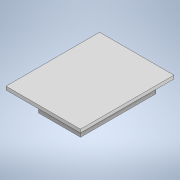
# Autodesk Inventor part: LCDScreen
Saved by Autodesk Inventor 2020 (Build 240168000, 168)
## iProperties
Created: 2019-07-11
Part Number: LCDScreen
Material: Generic
Document SubType Name: Modeling
Designer: El-KhouryJonathan
Density: 1 g/cm^3
Appearance: Default
Author: El-KhouryJonathan
Autodesk Inventor part; units mm, degrees
ref_plane "YZ Plane" through (0, 0, 0) normal (1, 0, 0) x (0, 1, 0)
ref_plane "XZ Plane" through (0, 0, 0) normal (0, 1, 0) x (-1, 0, 0)
ref_plane "XY Plane" through (0, 0, 0) normal (0, 0, 1) x (1, 0, 0)
sketch "Sketch1" plane through (0, 0, 0) normal (0, 1, 0) x (-1, 0, 0)
  point P0 (0, 0)
sketch "Sketch2" plane through (0, 0, 0) normal (0, 1, 0) x (-1, 0, 0)
  line L0 (-139.5, 175.3) -> (139.5, 175.3)
  line L1 (139.5, 175.3) -> (139.5, -175.3)
  line L2 (139.5, -175.3) -> (-139.5, -175.3)
  line L3 (-139.5, -175.3) -> (-139.5, 175.3)
  line L4 (-139.5, 175.3) -> (139.5, -175.3) construction
  line L5 (139.5, 175.3) -> (-139.5, -175.3) construction
  point P0 (0, 0)
  dimension "d0" = 350.6
  dimension "d1" = 279
  constraints: 12 end point, 2 midpoint, 2 parallel, 1 horizontal, 1 perpendicular
  measures "d0" distance of L0.end L1.end
  measures "d1" distance of L0.start L0.end
extrude "Extrusion1" add sketch "Sketch2" along normal blind 12.4
sketch "Sketch3" plane through (0, 0, 0) normal (0, -1, 0) x (1, 0, 0)
  line L0 (-125.5, -159.875) -> (125.5, -159.875)
  line L1 (125.5, -159.875) -> (125.5, 159.875)
  line L2 (125.5, 159.875) -> (-125.5, 159.875)
  line L3 (-125.5, 159.875) -> (-125.5, -159.875)
  line L4 (-125.5, -159.875) -> (125.5, 159.875) construction
  line L5 (125.5, -159.875) -> (-125.5, 159.875) construction
  point P0 (0, 0)
  dimension "d4" = 319.75
  dimension "d5" = 251
  constraints: 12 end point, 2 midpoint, 2 parallel, 1 horizontal, 1 perpendicular
  measures "d4" distance of L2.end L0.start
  measures "d5" distance of L1.end L2.end
extrude "Extrusion2" add sketch "Sketch3" along normal blind 13.5
sketch "Sketch4" plane through (0, -13.5, 0) normal (0, -1, 0) x (1, 0, 0)
  line L0 (125.5, 159.875) -> (-125.5, 159.875) projected
  line L1 (-125.5, 159.875) -> (-125.5, -159.875) projected
  line L2 (125.5, -159.875) -> (125.5, 159.875) projected
  line L3 (-125.5, -159.875) -> (125.5, -159.875) projected
  point P0 (0, 0)
  point P1 (-115.5, 149.875)
  point P2 (-115.5, -149.875)
  point P3 (115.5, 149.875)
  point P4 (115.5, -149.875)
  dimension "d15" = 10
  dimension "d16" = 10
  dimension "d19" = 299.75
  dimension "d22" = 231
  dimension "d25" = 10
  dimension "d26" = 10
  constraints: 1 horizontal, 1 vertical, 3 other
  measures "d15" distance from line of L0 point (-115.5, 149.875)
  measures "d16" distance from line of L1 point (-115.5, 149.875)
  measures "d19" distance of point (-115.5, 149.875) point (-115.5, -149.875)
  measures "d22" distance of point (-115.5, 149.875) point (115.5, 149.875)
  measures "d25" distance from line of L2 point (115.5, 149.875)
  measures "d26" distance from line of L3 point (-115.5, -149.875)
hole "Hole1" at (-115.5, -13.5, 149.875) at (115.5, -13.5, 149.875) at (115.5, -13.5, -149.875) at (-115.5, -13.5, -149.875) direction (0, 1, 0) diameter 9 depth 8 tip angle 118
sketch "Sketch5" plane through (0, -13.5, 0) normal (0, -1, 0) x (1, 0, 0)
  line L0 (125.5, 159.875) -> (-125.5, 159.875) projected
  line L1 (-125.5, 159.875) -> (-125.5, -159.875) projected
  line L2 (125.5, -159.875) -> (125.5, 159.875) projected
  point P0 (0, 0)
  point P1 (-115.5, 0)
  point P2 (115.5, 0)
  dimension "d34" = 159.875
  dimension "d35" = 10
  dimension "d38" = 231
  dimension "d43" = 10
  constraints: 1 horizontal, 1 other
  measures "d34" distance from line of point (-115.5, 0) L0
  measures "d35" distance from line of L1 point (-115.5, 0)
  measures "d38" distance of point (-115.5, 0) point (115.5, 0)
  measures "d43" distance from line of L2 point (115.5, 0)
hole "Hole2" at (-115.5, -13.5, 0) at (115.5, -13.5, 0) direction (0, 1, 0) diameter 9 depth 8 tip angle 118
sketch "Sketch6" plane through (0, -13.5, 0) normal (0, -1, 0) x (1, 0, 0)
  circle A0 centre (-115.5, 149.875) radius 4.5 projected
  line L0 (-125.5, 159.875) -> (-125.5, -159.875) projected
  line L1 (-125.5, -159.875) -> (125.5, -159.875) projected
  line L2 (125.5, 159.875) -> (-125.5, 159.875) projected
  point P0 (0, 0)
  point P1 (-1, 149.875)
  point P2 (-1, -149.875)
  dimension "d55" = 298
  dimension "d52" = 124.5
  dimension "d60" = 10
  dimension "d188" = 10
  constraints: 1 vertical, 1 other
  measures "d52" distance from line of L0 point (-1, 149.875)
  measures "d60" distance from line of L1 point (-1, -149.875)
  measures "d188" distance from line of L2 point (-1, 149.875)
hole "Hole3" at (-1, -13.5, -149.875) at (-1, -13.5, 149.875) direction (0, 1, 0) diameter 9 depth 8 tip angle 118
sketch "Sketch7" plane through (0, -13.5, 0) normal (0, -1, 0) x (1, 0, 0)
  line L0 (-51.5, 141.825) -> (106.5, 141.825)
  line L1 (106.5, 141.825) -> (106.5, -139.875)
  line L2 (106.5, -139.875) -> (-51.5, -139.875)
  line L3 (-51.5, -139.875) -> (-51.5, 141.825)
  line L4 (-51.5, 141.825) -> (106.5, -139.875) construction
  line L5 (106.5, 141.825) -> (-51.5, -139.875) construction
  line L6 (125.5, -159.875) -> (125.5, 159.875) projected
  line L7 (-125.5, -159.875) -> (125.5, -159.875) projected
  point P0 (0, 0)
  dimension "d61" = 281.7
  dimension "d62" = 158
  dimension "d63" = 19
  dimension "d64" = 20
  constraints: 12 end point, 2 parallel, 1 horizontal, 1 perpendicular
  measures "d61" distance of L2.end L0.start
  measures "d62" distance of L0.start L0.end
  measures "d63" distance between parallel lines of L6 L1
  measures "d64" distance between parallel lines of L7 L2
extrude "Extrusion3" add sketch "Sketch7" along normal blind 33.6
sketch "Sketch8" plane through (0, -47.1, 0) normal (0, -1, 0) x (1, 0, 0)
  line L0 (100.2, 131.825) -> (82.2, 131.825)
  line L1 (82.2, 131.825) -> (82.2, 15.825)
  line L2 (82.2, 15.825) -> (100.2, 15.825)
  line L3 (100.2, 15.825) -> (100.2, 131.825)
  line L4 (100.2, 131.825) -> (82.2, 15.825) construction
  line L5 (82.2, 131.825) -> (100.2, 15.825) construction
  line L6 (106.5, -139.875) -> (106.5, 141.825) projected
  line L7 (106.5, 141.825) -> (-51.5, 141.825) projected
  point P0 (0, 0)
  point P1 (91.2, 73.825)
  dimension "d67" = 116
  dimension "d68" = 18
  dimension "d69" = 6.3
  dimension "d70" = 10
  constraints: 12 end point, 2 midpoint, 2 parallel, 1 horizontal, 1 perpendicular
  measures "d67" distance of L0.end L1.end
  measures "d68" distance of L1.end L2.end
  measures "d69" distance between parallel lines of L6 L3
  measures "d70" distance between parallel lines of L7 L0
extrude "Extrusion4" add sketch "Sketch8" along normal blind 1
sketch "Sketch9" plane through (0, -47.1, 0) normal (0, -1, 0) x (1, 0, 0)
  line L0 (101, -70.275) -> (43.15, -70.275)
  line L1 (43.15, -70.275) -> (43.15, -128.125)
  line L2 (43.15, -128.125) -> (101, -128.125)
  line L3 (101, -128.125) -> (101, -70.275)
  line L4 (101, -70.275) -> (43.15, -128.125) construction
  line L5 (43.15, -70.275) -> (101, -128.125) construction
  line L6 (106.5, -139.875) -> (106.5, 141.825) projected
  line L7 (-51.5, -139.875) -> (106.5, -139.875) projected
  point P0 (0, 0)
  point P1 (72.075, -99.2)
  dimension "d73" = 5.5
  dimension "d74" = 57.85
  dimension "d75" = 11.75
  dimension "d76" = 57.85
  constraints: 12 end point, 2 midpoint, 2 parallel, 1 horizontal, 1 perpendicular
  measures "d73" distance between parallel lines of L3 L6
  measures "d74" distance of L2.end L0.start
  measures "d75" distance between parallel lines of L7 L2
  measures "d76" distance of L0.start L0.end
extrude "Extrusion5" add sketch "Sketch9" along normal blind 1
sketch "Sketch10" plane through (0, -47.1, 0) normal (0, -1, 0) x (1, 0, 0)
  line L0 (106.5, 141.825) -> (-51.5, 141.825) projected
  line L1 (-51.5, 141.825) -> (-51.5, -139.875) projected
  line L2 (-51.5, -139.875) -> (106.5, -139.875) projected
  point P0 (0, 0)
  point P1 (-44.5, 121.025)
  point P2 (-44.5, -119.075)
  dimension "d86" = 20.8
  dimension "d87" = 7
  dimension "d90" = 240.1
  dimension "d95" = 20.8
  constraints: 1 vertical, 1 other
  measures "d86" distance from line of L0 point (-44.5, 121.025)
  measures "d87" distance from line of L1 point (-44.5, 121.025)
  measures "d90" distance of point (-44.5, 121.025) point (-44.5, -119.075)
  measures "d95" distance from line of L2 point (-44.5, -119.075)
hole "Hole4" at (-44.5, -47.1, 121.025) at (-44.5, -47.1, -119.075) direction (0, 1, 0) diameter 7 depth 8 tip angle 118
sketch "Sketch11" plane through (0, -47.1, 0) normal (0, -1, 0) x (1, 0, 0)
  line L0 (106.5, 141.825) -> (-51.5, 141.825) projected
  line L1 (-51.5, 141.825) -> (-51.5, -139.875) projected
  line L2 (125.5, 159.875) -> (-125.5, 159.875) projected
  point P0 (0, 0)
  point P1 (-44.5, 0.825)
  dimension "d103" = 141
  dimension "d104" = 7
  dimension "d185" = 159.05
  measures "d103" distance from line of point (-44.5, 0.825) L0
  measures "d104" distance from line of L1 point (-44.5, 0.825)
  measures "d185" distance from line of point (-44.5, 0.825) L2
hole "Hole5" at (-44.5, -47.1, 0.825) direction (0, 1, 0) diameter 7 depth 8 tip angle 118
sketch "Sketch12" plane through (0, -47.1, 0) normal (0, -1, 0) x (1, 0, 0)
  line L0 (106.5, 141.825) -> (-51.5, 141.825) projected
  line L1 (-51.5, 141.825) -> (-51.5, -139.875) projected
  point P0 (0, 0)
  point P1 (-17.7, 38.475)
  point P2 (-17.7, -36.025)
  point P3 (56.8, 38.475)
  point P4 (56.8, -36.025)
  dimension "d112" = 103.35
  dimension "d113" = 33.8
  dimension "d116" = 74.5
  dimension "d119" = 74.5
  constraints: 1 horizontal, 1 vertical, 3 other
  measures "d112" distance from line of L0 point (-17.7, 38.475)
  measures "d113" distance from line of L1 point (-17.7, 38.475)
  measures "d116" distance of point (-17.7, 38.475) point (-17.7, -36.025)
  measures "d119" distance of point (-17.7, 38.475) point (56.8, 38.475)
hole "Hole6" at (-17.7, -47.1, 38.475) at (56.8, -47.1, 38.475) at (56.8, -47.1, -36.025) at (-17.7, -47.1, -36.025) direction (0, 1, 0) diameter 7 depth 8 tip angle 118
sketch "Sketch13" plane through (-51.5, -13.5, -139.875) normal (-1, 0, 0) x (0, 0, 1)
  line L0 (223, -27.9) -> (191.35, -27.9)
  line L1 (191.35, -27.9) -> (191.35, -8.5)
  line L2 (191.35, -8.5) -> (223, -8.5)
  line L3 (223, -8.5) -> (223, -27.9)
  line L4 (223, -27.9) -> (191.35, -8.5) construction
  line L5 (191.35, -27.9) -> (223, -8.5) construction
  line L6 (281.7, 0) -> (281.7, -33.6) projected
  line L7 (281.7, -33.6) -> (0, -33.6) projected
  point P0 (139.875, 13.5)
  point P1 (207.175, -18.2)
  dimension "d122" = 58.7
  dimension "d123" = 31.65
  dimension "d124" = 19.4
  dimension "d133" = 5.7
  constraints: 12 end point, 2 midpoint, 2 parallel, 1 horizontal, 1 perpendicular
  measures "d122" distance between parallel lines of L6 L3
  measures "d123" distance of L0.start L0.end
  measures "d124" distance of L0.end L1.end
  measures "d133" distance between parallel lines of L7 L0
extrude "Extrusion6" add sketch "Sketch13" along normal blind 1.5
sketch "Sketch14" plane through (-51.5, -13.5, -139.875) normal (-1, 0, 0) x (0, 0, 1)
  line L0 (139.25, -14.2) -> (122.25, -14.2)
  line L1 (122.25, -14.2) -> (122.25, -8)
  line L2 (122.25, -8) -> (139.25, -8)
  line L3 (139.25, -8) -> (139.25, -14.2)
  line L4 (139.25, -14.2) -> (122.25, -8) construction
  line L5 (122.25, -14.2) -> (139.25, -8) construction
  line L6 (191.35, -8.5) -> (191.35, -27.9) projected
  line L7 (281.7, -33.6) -> (0, -33.6) projected
  line L8 (191.35, -27.9) -> (223, -27.9) projected
  line L9 (299.75, 0) -> (-20, 0) projected
  line L10 (223, -8.5) -> (191.35, -8.5) projected
  point P0 (139.875, 13.5)
  point P1 (130.75, -11.1)
  dimension "d127" = 52.1
  dimension "d128" = 6.2
  dimension "d129" = 17
  dimension "d130" = 19.4
  dimension "d131" = 5.7
  dimension "d132" = 8.5
  constraints: 12 end point, 2 midpoint, 2 parallel, 1 horizontal, 1 perpendicular
  measures "d127" distance between parallel lines of L3 L6
  measures "d128" distance of L2.end L0.start
  measures "d129" distance of L0.start L0.end
  measures "d130" distance between parallel lines of L7 L0
  measures "d131" distance between parallel lines of L8 L7
  measures "d132" distance between parallel lines of L9 L10
extrude "Extrusion7" cut sketch "Sketch14" against normal blind 1.5
sketch "Sketch15" plane through (-51.5, -13.5, -139.875) normal (-1, 0, 0) x (0, 0, 1)
  line L0 (116.35, -14.2) -> (101.55, -14.2)
  line L1 (101.55, -14.2) -> (101.55, -8)
  line L2 (101.55, -8) -> (116.35, -8)
  line L3 (116.35, -8) -> (116.35, -14.2)
  line L4 (116.35, -14.2) -> (101.55, -8) construction
  line L5 (101.55, -14.2) -> (116.35, -8) construction
  line L6 (122.25, -14.2) -> (122.25, -8) projected
  line L7 (281.7, -33.6) -> (0, -33.6) projected
  point P0 (139.875, 13.5)
  point P1 (108.95, -11.1)
  dimension "d136" = 5.9
  dimension "d137" = 6.2
  dimension "d138" = 14.8
  dimension "d141" = 19.4
  constraints: 12 end point, 2 midpoint, 2 parallel, 1 horizontal, 1 perpendicular
  measures "d136" distance between parallel lines of L3 L6
  measures "d137" distance of L0.end L1.end
  measures "d138" distance of L0.start L0.end
  measures "d141" distance between parallel lines of L7 L0
extrude "Extrusion8" cut sketch "Sketch15" against normal blind 1.5
sketch "Sketch16" plane through (-51.5, -13.5, -139.875) normal (-1, 0, 0) x (0, 0, 1)
  circle A0 centre (90.05, -14.2) radius 2.5
  line L0 (101.55, -14.2) -> (101.55, -8) projected
  line L1 (281.7, -33.6) -> (0, -33.6) projected
  circle A1 centre (65.05, -14.2) radius 2.5
  point P0 (139.875, 13.5)
  dimension "d142" = 11.5
  dimension "d143" = 19.4
  dimension "d144" = 5
  dimension "d147" = 25
  constraints: 2 centre point, 1 horizontal, 2 other
  measures "d142" distance from line of A0.centre L0
  measures "d143" distance from line of L1 A0.centre
  measures "d144" diameter of A0
  measures "d147" distance of A0.centre A1.centre
extrude "Extrusion9" add sketch "Sketch16" along normal blind 5
sketch "Sketch17" plane through (-51.5, -13.5, -139.875) normal (-1, 0, 0) x (0, 0, 1)
  line L0 (86.05, -18.35) -> (70.65, -18.35)
  line L1 (70.65, -18.35) -> (70.65, -10.05)
  line L2 (70.65, -10.05) -> (86.05, -10.05)
  line L3 (86.05, -10.05) -> (86.05, -18.35)
  line L4 (86.05, -18.35) -> (70.65, -10.05) construction
  line L5 (70.65, -18.35) -> (86.05, -10.05) construction
  line L6 (101.55, -14.2) -> (101.55, -8) projected
  line L7 (281.7, -33.6) -> (0, -33.6) projected
  point P0 (139.875, 13.5)
  point P1 (78.35, -14.2)
  dimension "d154" = 8.3
  dimension "d155" = 15.4
  dimension "d156" = 15.5
  dimension "d157" = 19.4
  constraints: 12 end point, 2 midpoint, 2 parallel, 1 horizontal, 1 perpendicular
  measures "d154" distance of L2.end L0.start
  measures "d155" distance of L0.start L0.end
  measures "d156" distance between parallel lines of L3 L6
  measures "d157" distance from line of L7 point (78.35, -14.2)
extrude "Extrusion10" add sketch "Sketch17" along normal blind 5
sketch "Sketch18" plane through (0, -13.5, 0) normal (0, -1, 0) x (1, 0, 0)
  line L0 (125.5, 159.875) -> (-125.5, 159.875) projected
  line L1 (-125.5, 159.875) -> (-125.5, -159.875) projected
  line L2 (-125.5, -159.875) -> (125.5, -159.875) projected
  point P0 (0, 0)
  point P1 (-57.6, 117.025)
  point P2 (-57.6, -117.025)
  dimension "d167" = 42.85
  dimension "d168" = 67.9
  dimension "d171" = 234.05
  dimension "d176" = 42.85
  constraints: 1 vertical, 1 other
  measures "d167" distance from line of L0 point (-57.6, 117.025)
  measures "d168" distance from line of L1 point (-57.6, 117.025)
  measures "d171" distance of point (-57.6, 117.025) point (-57.6, -117.025)
  measures "d176" distance from line of L2 point (-57.6, -117.025)
hole "Hole7" at (-57.6, -13.5, 117.025) at (-57.6, -13.5, -117.025) direction (0, 1, 0) diameter 7 depth 8 tip angle 118
sketch "Sketch19" plane through (0, -13.5, 0) normal (0, -1, 0) x (1, 0, 0)
  circle A0 centre (-57.6, 117.025) radius 3.5 projected
  line L0 (125.5, 159.875) -> (-125.5, 159.875) projected
  line L1 (-125.5, 159.875) -> (-125.5, -159.875) projected
  point P0 (0, 0)
  point P1 (-57.6, 0.825)
  dimension "d186" = 159.05
  dimension "d187" = 67.9
  measures "d186" distance from line of point (-57.6, 0.825) L0
  measures "d187" distance from line of L1 point (-57.6, 0.825)
hole "Hole8" at (-57.6, -13.5, 0.825) direction (0, 1, 0) diameter 7 depth 8 tip angle 118
body "Solid1"
